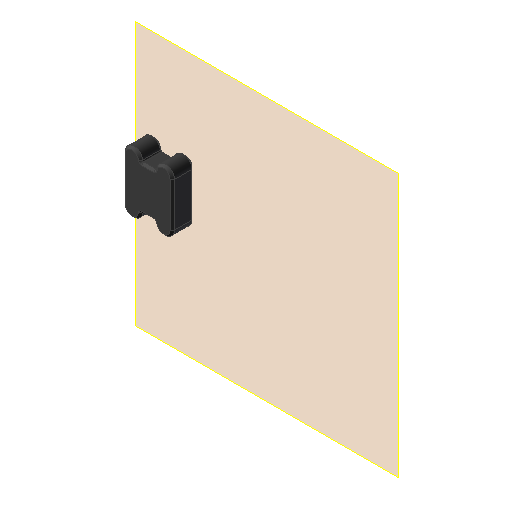
# Autodesk Inventor part: 10_Base_puzzle_nozzle_male_male
Saved by Autodesk Inventor 2025.1 (Build 291241020, 241B)
## iProperties
Created: 2023-05-17
Part Number: 10_Base_puzzle_nozzle_male_male
Material: Generisch
Document SubType Name: Modeling
Designer: diederichbenedict
Density: 1 g/cm^3
Appearance: Vorgabe
Description: not needed
Author: diederichbenedict
Autodesk Inventor part; units mm, degrees
ref_plane "YZ Plane" through (0, 0, 0) normal (1, 0, 0) x (0, 1, 0)
ref_plane "XZ Plane" through (0, 0, 0) normal (0, 1, 0) x (-1, 0, 0)
ref_plane "XY Plane" through (0, 0, 0) normal (0, 0, 1) x (1, 0, 0)
ref_plane "Arbeitsebene1" through (0, 0, 0) normal (0, 0, 1) x (1, 0, 0)
sketch "Skizze1" plane through (0, 0, 0) normal (0, 0, 1) x (1, 0, 0)
  line L0 (-2.5, -5) -> (27.5, -5) projected
  arc A0 (-5, -2.5) -> (-2.5, -5) centre (-2.5, -2.5) ccw projected
  line L1 (-5, 27.5) -> (-5, -2.5) projected
  arc A1 (-2.5, 30) -> (-5, 27.5) centre (-2.5, 27.5) ccw projected
  line L2 (27.5, 30) -> (-2.5, 30) projected
  arc A2 (30, 27.5) -> (27.5, 30) centre (27.5, 27.5) ccw projected
  line L3 (30, -2.5) -> (30, 27.5) projected
  arc A3 (27.5, -5) -> (30, -2.5) centre (27.5, -2.5) ccw projected
  circle A4 centre (12.5, -9.5) radius 4 projected
  line L4 (30.75, 28.4722) -> (33.3, 29.9445) projected
  line L5 (33.3, 29.9445) -> (35.85, 28.4722) projected
  line L6 (35.85, 28.4722) -> (35.85, 25.5278) projected
  line L7 (35.85, 25.5278) -> (33.3, 24.0555) projected
  line L8 (33.3, 24.0555) -> (30.75, 25.5278) projected
  line L9 (30.75, 25.5278) -> (30.75, 28.4722) projected
  line L10 (25.5278, 30.75) -> (24.0555, 33.3) projected
  line L11 (24.0555, 33.3) -> (25.5278, 35.85) projected
  line L12 (25.5278, 35.85) -> (28.4722, 35.85) projected
  line L13 (28.4722, 35.85) -> (29.9445, 33.3) projected
  line L14 (29.9445, 33.3) -> (28.4722, 30.75) projected
  line L15 (28.4722, 30.75) -> (25.5278, 30.75) projected
  line L16 (30.75, -3.4722) -> (33.3, -4.9445) projected
  line L17 (30.75, -0.5278) -> (30.75, -3.4722) projected
  line L18 (33.3, 0.9445) -> (30.75, -0.5278) projected
  line L19 (35.85, -0.5278) -> (33.3, 0.9445) projected
  line L20 (35.85, -3.4722) -> (35.85, -0.5278) projected
  line L21 (33.3, -4.9445) -> (35.85, -3.4722) projected
  line L22 (25.5278, -5.75) -> (24.0555, -8.3) projected
  line L23 (28.4722, -5.75) -> (25.5278, -5.75) projected
  line L24 (29.9445, -8.3) -> (28.4722, -5.75) projected
  line L25 (28.4722, -10.85) -> (29.9445, -8.3) projected
  line L26 (25.5278, -10.85) -> (28.4722, -10.85) projected
  line L27 (24.0555, -8.3) -> (25.5278, -10.85) projected
  line L28 (-5.75, 28.4722) -> (-8.3, 29.9445) projected
  line L29 (-5.75, 25.5278) -> (-5.75, 28.4722) projected
  line L30 (-8.3, 24.0555) -> (-5.75, 25.5278) projected
  line L31 (-10.85, 25.5278) -> (-8.3, 24.0555) projected
  line L32 (-10.85, 28.4722) -> (-10.85, 25.5278) projected
  line L33 (-8.3, 29.9445) -> (-10.85, 28.4722) projected
  line L34 (-0.5278, 30.75) -> (0.9445, 33.3) projected
  line L35 (-3.4722, 30.75) -> (-0.5278, 30.75) projected
  line L36 (-4.9445, 33.3) -> (-3.4722, 30.75) projected
  line L37 (-3.4722, 35.85) -> (-4.9445, 33.3) projected
  line L38 (-0.5278, 35.85) -> (-3.4722, 35.85) projected
  line L39 (0.9445, 33.3) -> (-0.5278, 35.85) projected
  line L40 (-0.5278, -5.75) -> (0.9445, -8.3) projected
  line L41 (0.9445, -8.3) -> (-0.5278, -10.85) projected
  line L42 (-0.5278, -10.85) -> (-3.4722, -10.85) projected
  line L43 (-3.4722, -10.85) -> (-4.9445, -8.3) projected
  line L44 (-4.9445, -8.3) -> (-3.4722, -5.75) projected
  line L45 (-3.4722, -5.75) -> (-0.5278, -5.75) projected
  line L46 (-5.75, -3.4722) -> (-8.3, -4.9445) projected
  line L47 (-8.3, -4.9445) -> (-10.85, -3.4722) projected
  line L48 (-10.85, -3.4722) -> (-10.85, -0.5278) projected
  line L49 (-10.85, -0.5278) -> (-8.3, 0.9445) projected
  line L50 (-8.3, 0.9445) -> (-5.75, -0.5278) projected
  line L51 (-5.75, -0.5278) -> (-5.75, -3.4722) projected
  circle A5 centre (-9.5, 12.5) radius 4 projected
  line L52 (36.5833, 6.6002) -> (37, 6.6003) projected
  arc A6 (31.3, 7.45) -> (36.5833, 6.6002) centre (34.01, 7.45) ccw projected
  line L53 (31.3, 17.55) -> (31.3, 7.45) projected
  arc A7 (36.5833, 18.3998) -> (31.3, 17.55) centre (34.01, 17.55) ccw projected
  line L54 (37, 18.3997) -> (36.5833, 18.3998) projected
  line L55 (37, 35.5) -> (37, 18.3997) projected
  arc A8 (37, 35.5) -> (35.5, 37) centre (35.5, 35.5) ccw projected
  line L56 (18.3997, 37) -> (35.5, 37) projected
  line L57 (18.3998, 36.5833) -> (18.3997, 37) projected
  arc A9 (17.55, 31.3) -> (18.3998, 36.5833) centre (17.55, 34.01) ccw projected
  line L58 (7.45, 31.3) -> (17.55, 31.3) projected
  arc A10 (6.6002, 36.5833) -> (7.45, 31.3) centre (7.45, 34.01) ccw projected
  line L59 (6.6003, 37) -> (6.6002, 36.5833) projected
  line L60 (-10.5, 37) -> (6.6003, 37) projected
  arc A11 (-10.5, 37) -> (-12, 35.5) centre (-10.5, 35.5) ccw projected
  line L61 (-12, 17) -> (-12, 35.5) projected
  line L62 (-13.8639, 17) -> (-12, 17) projected
  arc A12 (-14.6093, 17.6667) -> (-13.8639, 17) centre (-13.8639, 17.75) ccw projected
  arc A13 (-14.6093, 17.6667) -> (-17.6, 17.5) centre (-16.1, 17.5) ccw projected
  line L63 (-17.6, 7.5) -> (-17.6, 17.5) projected
  arc A14 (-17.6, 7.5) -> (-14.6093, 7.3333) centre (-16.1, 7.5) ccw projected
  arc A15 (-13.8639, 8) -> (-14.6093, 7.3333) centre (-13.8639, 7.25) ccw projected
  line L64 (-12, 8) -> (-13.8639, 8) projected
  line L65 (-12, -10.5) -> (-12, 8) projected
  arc A16 (-12, -10.5) -> (-10.5, -12) centre (-10.5, -10.5) ccw projected
  line L66 (8, -12) -> (-10.5, -12) projected
  line L67 (8, -13.8639) -> (8, -12) projected
  arc A17 (7.3333, -14.6093) -> (8, -13.8639) centre (7.25, -13.8639) ccw projected
  arc A18 (7.3333, -14.6093) -> (7.5, -17.6) centre (7.5, -16.1) ccw projected
  line L68 (17.5, -17.6) -> (7.5, -17.6) projected
  arc A19 (17.5, -17.6) -> (17.6667, -14.6093) centre (17.5, -16.1) ccw projected
  arc A20 (17, -13.8639) -> (17.6667, -14.6093) centre (17.75, -13.8639) ccw projected
  line L69 (17, -12) -> (17, -13.8639) projected
  line L70 (35.5, -12) -> (17, -12) projected
  arc A21 (35.5, -12) -> (37, -10.5) centre (35.5, -10.5) ccw projected
  line L71 (37, 6.6003) -> (37, -10.5) projected
  arc A22 (-18.1, 7.5) -> (-14.1124, 7.2778) centre (-16.1, 7.5) ccw projected
  arc A23 (-13.8639, 7.5) -> (-14.1124, 7.2778) centre (-13.8639, 7.25) ccw projected
  line L72 (-18.1, 17.5) -> (-18.1, 7.5) projected
  line L73 (-12, 8) -> (-13.8639, 8) projected
  line L74 (-13.8639, 7.5) -> (-13.8639, 8) projected
  line L75 (-13.8639, 7.5) -> (-12.5, 7.5) projected
  line L76 (-12, 8) -> (-12.5, 7.5) projected
  arc A24 (-14.1124, 17.7222) -> (-18.1, 17.5) centre (-16.1, 17.5) ccw projected
  line L77 (-12.5, 17.5) -> (-13.8639, 17.5) projected
  arc A25 (-14.1124, 17.7222) -> (-13.8639, 17.5) centre (-13.8639, 17.75) ccw projected
  line L78 (-12.5, 17.5) -> (-12.5, 7.5)
  point P0 (0, 0)
  constraints: 2 end point, 1 vertical
extrude "Extrusion1" add sketch "Skizze1" along normal blind 5 contours L78 A5 | A5 L78 L64 A15 A14 L63 A13 A12 L62 | L62 A12 A13 L63 A14 A15 L74 A23 A22 L72 A24 A25 L77 L78 | L78 L75 L74 L64 picked at (-12.6815, 11.8821)
mirror "Spiegeln1" about plane through (-12.5, 7.5, 0) normal (1, 0, 0) of "Extrusion1"
chamfer "Fase1" distance 0.5 angle 45 24 edges at (-8.7887, 19.4969, 5) (-6.9, 12.5, 5) (-8.7887, 5.5031, 5) (-10.9694, 7.4363, 5) (-12.5, 7.5, 5) (-14.0306, 7.4363, 5) (-16.2113, 5.5031, 5) (-18.1, 12.5, 5) (-16.2113, 19.4969, 5) (-14.0306, 17.5637, 5) (-12.5, 17.5, 5) (-10.9694, 17.5637, 5) (-12.5, 7.5, 0) (-10.9694, 7.4363, 0) (-8.7887, 5.5031, 0) (-6.9, 12.5, 0) (-8.7887, 19.4969, 0) (-10.9694, 17.5637, 0) (-12.5, 17.5, 0) (-14.0306, 17.5637, 0) (-16.2113, 19.4969, 0) (-18.1, 12.5, 0) (-16.2113, 5.5031, 0) (-14.0306, 7.4363, 0)
